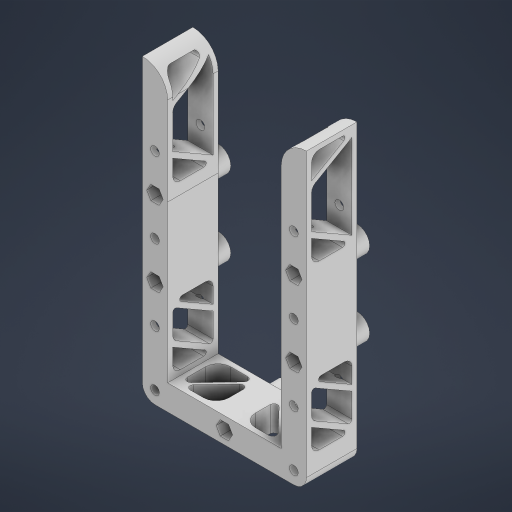
# Autodesk Inventor part: middle spacer
Saved by Autodesk Inventor 2023 (Build 270158000, 158)
## iProperties
Created: 2022-05-30
Part Number: middle spacer
Material: Generic
Document SubType Name: Modeling
Designer: vibhu
Density: 1 g/cm^3
Appearance: Default
Author: vibhu
Autodesk Inventor part; units mm, degrees
ref_plane "Work Plane3" through (0, 0, 0) normal (0, 0, 1) x (1, 0, 0)
ref_plane "Work Plane4" through (49.393398, 49.393398, 36.5) normal (0, 0, 1) x (0.7071068, 0.7071068, 0)
ref_plane "Work Plane5" through (0, 0, 0) normal (0, 0, 1) x (1, 0, 0)
ref_plane "Work Plane6" through (0, 0, 0) normal (0, 0, 1) x (1, 0, 0)
sketch "Sketch6" plane through (0, 0, 0) normal (0, 0, 1) x (1, 0, 0)
  circle A0 centre (0, -52) radius 1.75
  circle A1 centre (27.5, 15) radius 1.75
  circle A2 centre (27.5, -15) radius 1.75
  circle A3 centre (-27.5, -15) radius 1.75
  circle A4 centre (-27.5, 15) radius 1.75
  line L0 (12.5, 88) -> (-12.5, 88)
  circle A5 centre (27.5, -15) radius 5
  circle A6 centre (27.5, 15) radius 5
  circle A7 centre (-27.5, 15) radius 5
  circle A8 centre (-27.5, -15) radius 5
  circle A9 centre (0, -52) radius 5
  circle A10 centre (27.5, -15) radius 3.25 construction
  circle A11 centre (27.5, 15) radius 3.25 construction
  circle A12 centre (-27.5, 15) radius 3.25 construction
  circle A13 centre (-27.5, -15) radius 3.25 construction
  circle A14 centre (0, -52) radius 3.25 construction
  line L1 (22.5, -15) -> (22.5, -47)
  line L2 (22.5, -47) -> (-0.000001, -47)
  line L3 (32.5, -15) -> (32.5, -57)
  line L4 (32.5, -57) -> (-0.000001, -57)
  line L5 (0, -57) -> (-32.5, -57)
  line L6 (-32.5, -57) -> (-32.5, -15)
  line L7 (-22.5, -15) -> (-22.5, -47)
  line L8 (-22.5, -47) -> (-0.000001, -47)
  line L9 (32.5, -15) -> (32.5, 14.999999)
  line L10 (22.5, 15.000001) -> (22.5, -15)
  line L11 (-22.5, 15) -> (-22.5, -15)
  line L12 (-32.5, -15.000001) -> (-32.5, 15)
  point P0 (0, 0)
  dimension "d38" = 10
  dimension "d39" = 6.5
  dimension "d41" = 10
  constraints: 26 end point, 16 point on circle, 14 centre point, 10 coincident, 8 equal radius, 5 collinear, 5 parallel, 5 perpendicular, 3 vertical, 2 point on line, 2 tangent, 1 horizontal, 1 vertical alignment, 10 other
  measures "d38" diameter of A5
  measures "d39" diameter of A10
  measures "d41" distance between parallel lines of L4 L2
extrude "Extrusion3" add sketch "Sketch6" along normal blind 5 contours A5 | A6 | A9 | A8 | A7
sketch "Sketch7" plane through (0, -52, 5) normal (0, 0, 1) x (1, 0, 0)
  line L0 (22.5, 37) -> (22.5, 5)
  line L1 (32.5, 37) -> (32.5, -5)
  line L2 (22.5, 5) -> (-0.000001, 5)
  line L3 (32.5, -5) -> (-0.000001, -5)
  circle A0 centre (0, 0) radius 5
  circle A1 centre (-27.5, 37) radius 5
  line L4 (-22.5, 37) -> (-22.5, 5)
  line L5 (-32.5, -5) -> (-32.5, 37)
  line L6 (-22.5, 5) -> (-0.000001, 5)
  line L7 (0, -5) -> (-32.5, -5)
  circle A2 centre (27.5, 37) radius 5
  line L8 (32.5, 37) -> (32.5, 66.999999)
  line L9 (22.5, 67.000001) -> (22.5, 37)
  line L10 (-22.5, 67) -> (-22.5, 37)
  line L11 (-32.5, 36.999999) -> (-32.5, 67)
  circle A3 centre (-27.5, 67) radius 5
  circle A4 centre (27.5, 67) radius 5
  line L12 (32.5, 66.999999) -> (32.5, 111.999999)
  line L13 (22.500008, 102.000009) -> (22.5, 67.000001)
  circle A5 centre (27.5, 67) radius 5
  line L14 (-22.5, 66.999999) -> (-22.499992, 102.000009)
  line L15 (-32.5, 112.000019) -> (-32.5, 67)
  arc A6 (32.5, 111.999999) -> (22.500008, 102.000009) centre (32.5, 102.000007) ccw
  arc A7 (-22.499992, 102.000009) -> (-32.5, 112.000019) centre (-32.5, 102.000011) ccw
  point P0 (0, 52)
  dimension "d71" = 45
  constraints: 8 end point, 5 point on circle, 5 tangent, 2 centre point, 2 line through centre, 2 vertical, 1 horizontal alignment, 1 parallel
  measures "d71" distance of L8.end L12.end
extrude "Extrusion4" add sketch "Sketch7" along normal blind 20 contours A2 L1 L3 A0 L2 L0 | L9 A4 L8 A2 | L13 A6 L12 A4 | A0 L7 L5 A1 L4 L6 | A1 L11 A3 L10 | A3 L15 A7 L14
sketch "Sketch8" plane through (0, 0, 5) normal (0, 0, 1) x (1, 0, 0)
  arc A0 (27.5, -15) -> (27.5, -15) centre (27.5, -15) ccw
  arc A1 (27.5, -15) -> (27.5, -15) centre (27.5, -15) ccw
  arc A2 (0, -57) -> (-0.000001, -47) centre (0, -52) ccw
  arc A3 (-0.000001, -47) -> (0, -57) centre (0, -52) ccw
  circle A4 centre (0, -52) radius 1.75 construction
  arc A5 (32.5, -15) -> (22.5, -15) centre (27.5, -15) ccw
  arc A6 (22.5, -15) -> (32.5, -15) centre (27.5, -15) ccw
  circle A7 centre (27.5, -15) radius 1.75 construction
  arc A8 (32.5, 15) -> (22.5, 15.000001) centre (27.5, 15) ccw
  arc A9 (22.5, 15.000001) -> (32.5, 15) centre (27.5, 15) ccw
  circle A10 centre (27.5, 15) radius 1.75 construction
  arc A11 (-22.5, 15) -> (-32.5, 15) centre (-27.5, 15) ccw
  arc A12 (-32.5, 15) -> (-22.5, 15) centre (-27.5, 15) ccw
  circle A13 centre (-27.5, 15) radius 1.75 construction
  arc A14 (-27.5, -15) -> (-27.5, -15) centre (-27.5, -15) ccw
  arc A15 (-22.5, -15) -> (-32.5, -15) centre (-27.5, -15) ccw
  arc A16 (-32.5, -15) -> (-22.5, -15) centre (-27.5, -15) ccw
  circle A17 centre (-27.5, -15) radius 1.75 construction
  circle A18 centre (27.5, -15) radius 3.25 construction
  circle A19 centre (27.5, 15) radius 3.25 construction
  circle A20 centre (-27.5, 15) radius 3.25 construction
  circle A21 centre (-27.5, -15) radius 3.25 construction
  circle A22 centre (0, -52) radius 3.25 construction
  line L0 (25.875, -17.814583) -> (29.125, -17.814583)
  line L1 (-1.625, -54.814583) -> (1.625, -54.814583)
  line L2 (-29.125, -17.814583) -> (-25.875, -17.814583)
  line L3 (-29.125, 12.185417) -> (-25.875, 12.185417)
  line L4 (25.875, 12.185417) -> (29.125, 12.185417)
  line L5 (29.125, -17.814583) -> (30.75, -15)
  line L6 (30.75, -15) -> (29.125, -12.185417)
  line L7 (29.125, -12.185417) -> (25.875, -12.185417)
  line L8 (25.875, -12.185417) -> (24.25, -15)
  line L9 (24.25, -15) -> (25.875, -17.814583)
  line L10 (1.625, -54.814583) -> (3.25, -52)
  line L11 (3.25, -52) -> (1.625, -49.185417)
  line L12 (1.625, -49.185417) -> (-1.625, -49.185417)
  line L13 (-1.625, -49.185417) -> (-3.25, -52)
  line L14 (-3.25, -52) -> (-1.625, -54.814583)
  line L15 (-25.875, -17.814583) -> (-24.25, -15)
  line L16 (-24.25, -15) -> (-25.875, -12.185417)
  line L17 (-25.875, -12.185417) -> (-29.125, -12.185417)
  line L18 (-29.125, -12.185417) -> (-30.75, -15)
  line L19 (-30.75, -15) -> (-29.125, -17.814583)
  line L20 (-25.875, 12.185417) -> (-24.25, 15)
  line L21 (-24.25, 15) -> (-25.875, 17.814583)
  line L22 (-25.875, 17.814583) -> (-29.125, 17.814583)
  line L23 (-29.125, 17.814583) -> (-30.75, 15)
  line L24 (-30.75, 15) -> (-29.125, 12.185417)
  line L25 (29.125, 12.185417) -> (30.75, 15)
  line L26 (30.75, 15) -> (29.125, 17.814583)
  line L27 (29.125, 17.814583) -> (25.875, 17.814583)
  line L28 (25.875, 17.814583) -> (24.25, 15)
  line L29 (24.25, 15) -> (25.875, 12.185417)
  point P0 (0, 0)
  point P1 (25, -10.669873)
  point P2 (25, -19.330127)
  point P3 (32.116931, -16.919362)
  point P4 (32.116931, -13.080638)
  point P5 (-32.116931, -13.080638)
  point P6 (-32.116931, -16.919362)
  point P7 (1.625, -49.185417)
  point P8 (1.625, -54.814583)
  point P9 (32.116931, -16.919362)
  point P10 (-32.5, -15)
  dimension "d46" = 6.5
  dimension "d49" = 360
  dimension "d53" = 360
  dimension "d57" = 360
  dimension "d61" = 360
  dimension "d65" = 360
  constraints: 60 end point, 10 coincident, 10 point on circle, 5 centre point, 4 equal radius, 4 horizontal, 1 collinear, 98 other
  measures "d46" diameter of A18
sketch "Sketch8 outline for Extrusion5" plane through (0, 0, 5) normal (0, 0, 1) x (1, 0, 0)
  circle A0 centre (27.5, 15) radius 5
  line L0 (25.875, 12.185417) -> (24.25, 15)
  line L1 (24.25, 15) -> (25.875, 17.814583)
  line L2 (25.875, 17.814583) -> (29.125, 17.814583)
  line L3 (29.125, 17.814583) -> (30.75, 15)
  line L4 (30.75, 15) -> (29.125, 12.185417)
  line L5 (29.125, 12.185417) -> (25.875, 12.185417)
  circle A1 centre (-27.5, 15) radius 5
  line L6 (-29.125, 12.185417) -> (-30.75, 15)
  line L7 (-30.75, 15) -> (-29.125, 17.814583)
  line L8 (-29.125, 17.814583) -> (-25.875, 17.814583)
  line L9 (-25.875, 17.814583) -> (-24.25, 15)
  line L10 (-24.25, 15) -> (-25.875, 12.185417)
  line L11 (-25.875, 12.185417) -> (-29.125, 12.185417)
  circle A2 centre (-27.5, -15) radius 5
  line L12 (-29.125, -17.814583) -> (-30.75, -15)
  line L13 (-30.75, -15) -> (-29.125, -12.185417)
  line L14 (-29.125, -12.185417) -> (-25.875, -12.185417)
  line L15 (-25.875, -12.185417) -> (-24.25, -15)
  line L16 (-24.25, -15) -> (-25.875, -17.814583)
  line L17 (-25.875, -17.814583) -> (-29.125, -17.814583)
  circle A3 centre (0, -52) radius 5
  line L18 (-1.625, -54.814583) -> (-3.25, -52)
  line L19 (-3.25, -52) -> (-1.625, -49.185417)
  line L20 (-1.625, -49.185417) -> (1.625, -49.185417)
  line L21 (1.625, -49.185417) -> (3.25, -52)
  line L22 (3.25, -52) -> (1.625, -54.814583)
  line L23 (1.625, -54.814583) -> (-1.625, -54.814583)
  circle A4 centre (27.5, -15) radius 5
  line L24 (25.875, -17.814583) -> (24.25, -15)
  line L25 (24.25, -15) -> (25.875, -12.185417)
  line L26 (25.875, -12.185417) -> (29.125, -12.185417)
  line L27 (29.125, -12.185417) -> (30.75, -15)
  line L28 (30.75, -15) -> (29.125, -17.814583)
  line L29 (29.125, -17.814583) -> (25.875, -17.814583)
extrude "Extrusion5" add sketch "Sketch8 outline for Extrusion5" along normal up to surface (20 mm away)
fillet "Fillet1" radius 5 2 edges at (-32.5, -57, 15) (32.5, -57, 15)
sketch "Sketch9" plane through (0, -52, 25) normal (0, 0, 1) x (1, 0, 0)
  circle A0 centre (27.5, 52) radius 1.75
  circle A1 centre (-27.5, 52) radius 1.75
  circle A2 centre (27.5, 37) radius 1.75 construction
  circle A3 centre (-27.5, 37) radius 1.75 construction
  circle A4 centre (27.5, 0) radius 1.75
  circle A5 centre (-27.5, 0) radius 1.75
  circle A6 centre (0, 0) radius 1.75 construction
  point P0 (0, 52)
  constraints: 4 centre point, 4 equal radius, 4 horizontal alignment, 4 vertical alignment
extrude "Extrusion6" cut sketch "Sketch9" against normal up to surface (20 mm away)
sketch "Sketch10" plane through (0, -52, 5) normal (0, 0, -1) x (-1, 0, 0)
  circle A0 centre (-27.5, 52) radius 1.75
  circle A1 centre (27.5, 52) radius 1.75
  circle A2 centre (27.5, 0) radius 1.75
  circle A3 centre (-27.5, 52) radius 3.25 construction
  circle A4 centre (27.5, 52) radius 3.25 construction
  circle A5 centre (27.5, 0) radius 1.75
  circle A6 centre (27.5, 0) radius 3.25 construction
  circle A7 centre (-27.5, 0) radius 1.75
  circle A8 centre (-27.5, 0) radius 3.25 construction
  line L0 (-25.875, 2.814583) -> (-29.125, 2.814583)
  line L1 (-25.875, 49.185417) -> (-29.125, 49.185417)
  line L2 (29.125, 49.185417) -> (25.875, 49.185417)
  line L3 (29.125, -2.814583) -> (25.875, -2.814583)
  line L4 (-29.125, 2.814583) -> (-30.75, 0)
  line L5 (-30.75, 0) -> (-29.125, -2.814583)
  line L6 (-29.125, -2.814583) -> (-25.875, -2.814583)
  line L7 (-25.875, -2.814583) -> (-24.25, 0)
  line L8 (-24.25, 0) -> (-25.875, 2.814583)
  line L9 (30.75, 0) -> (29.125, -2.814583)
  line L10 (29.125, 2.814583) -> (30.75, 0)
  line L11 (25.875, 2.814583) -> (29.125, 2.814583)
  line L12 (24.25, 0) -> (25.875, 2.814583)
  line L13 (25.875, -2.814583) -> (24.25, 0)
  line L14 (30.75, 52) -> (29.125, 49.185417)
  line L15 (29.125, 54.814583) -> (30.75, 52)
  line L16 (25.875, 54.814583) -> (29.125, 54.814583)
  line L17 (24.25, 52) -> (25.875, 54.814583)
  line L18 (25.875, 49.185417) -> (24.25, 52)
  line L19 (-24.25, 52) -> (-25.875, 49.185417)
  line L20 (-25.875, 54.814583) -> (-24.25, 52)
  line L21 (-29.125, 54.814583) -> (-25.875, 54.814583)
  line L22 (-30.75, 52) -> (-29.125, 54.814583)
  line L23 (-29.125, 49.185417) -> (-30.75, 52)
  point P0 (0, 52)
  point P1 (-25.875, 2.814583)
  point P2 (-29.125, 2.814583)
  point P3 (-30.75, 0)
  point P4 (29.125, -2.814583)
  point P5 (30.75, 0)
  point P6 (29.125, 2.814583)
  point P7 (24.25, 0)
  point P8 (25.875, -2.814583)
  dimension "d74" = 6.5
  dimension "d77" = 360
  dimension "d81" = 360
  dimension "d85" = 360
  dimension "d89" = 360
  constraints: 48 end point, 8 coincident, 8 point on circle, 4 centre point, 3 equal length, 3 equal radius, 1 horizontal, 76 other
  measures "d74" diameter of A3
extrude "Extrusion7" cut sketch "Sketch10" against normal blind 3
sketch "Sketch11" plane through (0, -52, 25) normal (0, 0, 1) x (1, 0, 0)
  circle A0 centre (27.5, 82) radius 1.75
  circle A1 centre (-27.5, 82) radius 1.75
  circle A2 centre (-27.5, 22) radius 1.75
  circle A3 centre (27.5, 22) radius 1.75
  circle A4 centre (27.5, 37) radius 1.75 projected
  circle A5 centre (-27.5, 37) radius 1.75 projected
  point P0 (0, 52)
  dimension "d93" = 3.5
  dimension "d94" = 30
  dimension "d95" = 30
  constraints: 4 centre point, 4 vertical alignment, 3 equal radius, 2 horizontal alignment
  measures "d93" diameter of A3
  measures "d94" vertical distance of point (0, 52) A0.centre
  measures "d95" vertical distance of A3.centre point (0, 52)
extrude "Extrusion8" cut sketch "Sketch11" against normal up to surface (20 mm away) contours A0 | A1 | A2 | A3
sketch "Sketch12" plane through (0, -57, 5) normal (0, -1, 0) x (1, 0, 0)
  line L0 (-20.5, 2) -> (-20.5, 18)
  line L1 (-20.5, 18) -> (-5.25, 2)
  line L2 (-5.25, 2) -> (-20.5, 2)
  line L3 (-22.5, 0) -> (-22.5, 20) construction
  line L4 (-1.625, 20) -> (1.625, 20) construction
  line L5 (0, 20) -> (0, -13.018808) construction
  line L6 (-3.25, 0) -> (-3.25, 20) construction
  line L7 (-27.5, 20) -> (27.5, 20)
  line L8 (-27.5, 0) -> (0, 0)
  line L9 (-5.25, 3.449407) -> (-19.118534, 18)
  line L10 (-19.118534, 18) -> (-5.25, 18)
  line L11 (-5.25, 18) -> (-5.25, 3.449407)
  line L12 (20.5, 2) -> (20.5, 18)
  line L13 (20.5, 18) -> (5.25, 2)
  line L14 (5.25, 2) -> (20.5, 2)
  line L15 (5.25, 3.449407) -> (19.118534, 18)
  line L16 (19.118534, 18) -> (5.25, 18)
  line L17 (5.25, 18) -> (5.25, 3.449407)
  point P0 (0, -5)
  dimension "d98" = 2
  dimension "d99" = 2
  dimension "d100" = 2
  dimension "d101" = 2
  dimension "d103" = 1
  constraints: 26 end point, 6 symmetric about line, 2 perpendicular, 2 vertical, 1 horizontal, 1 horizontal alignment, 1 midpoint, 1 parallel, 1 vertical alignment
  measures "d98" distance between parallel lines of L3 L0
  measures "d99" distance from line of L6 L1.end
  measures "d100" distance from line of L7 L0.end
  measures "d101" distance between parallel lines of L8 L2
  measures "d103" distance between parallel lines of L9 L1
extrude "Extrusion9" cut sketch "Sketch12" against normal up to surface (10 mm away)
fillet "Fillet2" radius 5 4 edges at (-20.5, -52, 7) (-5.25, -52, 23) (20.5, -52, 7) (5.25, -52, 23)
fillet "Fillet3" radius 1.5 8 edges at (-20.5, -52, 23) (-5.25, -52, 8.4494) (-5.25, -52, 7) (-19.1185, -52, 23) (20.5, -52, 23) (19.1185, -52, 23) (5.25, -52, 7) (5.25, -52, 8.4494)
sketch "Sketch13" plane through (32.5, 15, 5) normal (1, 0, 0) x (0, 0, -1)
  line L0 (-18, -60) -> (-2, -60)
  line L1 (-2, -60) -> (-18, -50.762396)
  line L2 (-18, -50.762396) -> (-18, -60)
  line L3 (-2, -57.690599) -> (-18, -48.452995)
  line L4 (-18, -48.452995) -> (-18, -37.123984)
  line L5 (-18, -37.123984) -> (-2, -46.361588)
  line L6 (-2, -46.361588) -> (-2, -57.690599)
  line L7 (-2, -44.052187) -> (-18, -34.814583)
  line L8 (-18, -34.814583) -> (-2, -34.814583)
  line L9 (-2, -34.814583) -> (-2, -44.052187)
  line L10 (-20, -67) -> (-20, 44.999999)
  line L11 (0, -67) -> (0, -30)
  line L12 (0, -62) -> (-20, -62)
  line L13 (0, -32.814583) -> (-20, -32.814583)
  line L14 (-18, 4.814583) -> (-2, 4.814583)
  line L15 (-2, 4.814583) -> (-18, 14.052187)
  line L16 (-18, 14.052187) -> (-18, 4.814583)
  line L17 (0, 2.814583) -> (-20, 2.814583)
  line L18 (-2, 7.123984) -> (-18, 16.361588)
  line L19 (-18, 16.361588) -> (-18, 31.452994)
  line L20 (-18, 31.452994) -> (-2, 40.690598)
  line L21 (-2, 40.690598) -> (-2, 7.123984)
  line L22 (-18, 33.762395) -> (-2, 42.999999)
  line L23 (-2, 42.999999) -> (-18, 42.999999)
  line L24 (-18, 42.999999) -> (-18, 33.762395)
  line L25 (0, 44.999999) -> (-20, 44.999999)
  point P0 (5, -15)
  point P1 (-10, -39.433385)
  dimension "d108" = 2
  dimension "d109" = 2
  dimension "d110" = 30
  dimension "d111" = 2
  dimension "d112" = 2
  dimension "d113" = 2
  dimension "d114" = 2
  dimension "d117" = 2
  dimension "d119" = 30
  dimension "d120" = 2
  dimension "d121" = 2
  dimension "d122" = 30
  dimension "d123" = 2
  constraints: 40 end point, 10 vertical alignment, 6 parallel, 5 vertical, 4 perpendicular, 2 horizontal, 2 point on line, 1 midpoint
  measures "d108" distance between parallel lines of L2 L10
  measures "d109" distance between parallel lines of L11 L6
  measures "d110" angle of L1 L0
  measures "d111" distance between parallel lines of L3 L1
  measures "d112" distance from line of point (-10, -39.433) L5
  measures "d113" distance between parallel lines of L12 L0
  measures "d114" distance between parallel lines of L13 L8
  measures "d117" distance between parallel lines of L14 L17
  measures "d119" angle of L15 L14
  measures "d120" distance between parallel lines of L15 L18
  measures "d121" distance between parallel lines of L22 L20
  measures "d122" angle of L22 L23
  measures "d123" distance between parallel lines of L25 L23
extrude "Extrusion10" cut sketch "Sketch13" against normal up to surface (65 mm away) contours L2 L1 L0 | L3 L4 L5 L6 | L7 L8 L9 | L16 L15 L14 | L18 L19 L20 L21 | L24 L23 L22
fillet "Fillet4" radius 3 8 edges at (27.5, -19.8146, 7) (27.5, -45, 23) (-27.5, -45, 23) (-27.5, -19.8146, 7) (-27.5, 19.8146, 23) (27.5, 19.8146, 23) (29.5, 58, 23) (-29.5, 58, 23)
fillet "Fillet5" radius 3 4 edges at (27.5, -33.453, 23) (-27.5, -33.453, 23) (-27.5, 46.453, 23) (27.5, 46.453, 23)
fillet "Fillet6" radius 1 12 edges at (27.5, -22.124, 23) (27.5, -42.6906, 7) (-27.5, -42.6906, 7) (-27.5, -22.124, 23) (-27.5, 19.8146, 7) (27.5, 19.8146, 7) (29.5, 58, 7) (-29.5, 58, 7) (27.5, -45, 7) (27.5, -19.8146, 23) (-27.5, -19.8146, 23) (-27.5, -45, 7)
body "Solid2"
